# Autodesk Inventor part: DEVICE?
Saved by Autodesk Inventor 2015 SP1 (Build 190203100, 203)
## iProperties
Created: 2015-06-25
Part Number: DEVICE?
Material: Generic
Document SubType Name: Modeling
Designer: Patrick
Density: 1 g/cm^3
Appearance: TOOL_HOLE, DEVICE_
Author: Patrick
Autodesk Inventor part; units mm, degrees
ref_plane "YZ Plane" through (0, 0, 0) normal (1, 0, 0) x (0, 1, 0)
ref_plane "XZ Plane" through (0, 0, 0) normal (0, 1, 0) x (-1, 0, 0)
ref_plane "XY Plane" through (0, 0, 0) normal (0, 0, 1) x (1, 0, 0)
sketch "TOOL_HOLE, DEVICE__1" plane through (0, 0, 0) normal (0, 0, 1) x (1, 0, 0)
  line L0 (-1.5, -1.5) -> (-1.5, 1.5)
  line L1 (-1.5, 1.5) -> (1.5, 1.5)
  line L2 (1.5, 1.5) -> (1.5, -1.5)
  line L3 (1.5, -1.5) -> (-1.5, -1.5)
  constraints: 8 end point
extrude "Extrusion1" add sketch "TOOL_HOLE, DEVICE__1" along normal blind 1
body "Solid1"
